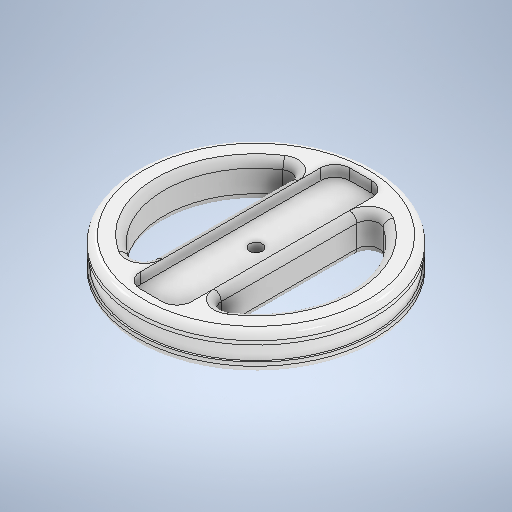
# Autodesk Inventor part: roue
Saved by Autodesk Inventor 2025 (Build 290162000, 162)
## iProperties
Created: 2024-09-05
Part Number: roue
Material: Générique
Document SubType Name: Modeling
Designer: chass
Density: 1 g/cm^3
Appearance: Par défaut
Author: chass
## iProperties of the stored document roue_Impression 3D.ipt
Created: 2024-09-05
Part Number: roue_Impression 3D
Material: Générique
Document SubType Name: Modeling
Designer: chass
Density: 1 g/cm^3
Appearance: Par défaut
Author: chass
Autodesk Inventor part; units mm, degrees
ref_plane "YZ Plane" through (0, 0, 0) normal (1, 0, 0) x (0, 1, 0)
ref_plane "XZ Plane" through (0, 0, 0) normal (0, 1, 0) x (-1, 0, 0)
ref_plane "XY Plane" through (0, 0, 0) normal (0, 0, 1) x (1, 0, 0)
sketch "Esquisse2" plane through (0, 0, 0) normal (0, 0, 1) x (1, 0, 0)
  line L0 (0, 0) -> (32.5, 0)
  line L1 (32.5, 0) -> (32.5, -10)
  line L2 (32.5, -10) -> (0, -10)
  line L3 (0, -10) -> (0, 0)
  line L4 (32.5, -3) -> (32, -3)
  line L5 (32, -3) -> (32, -7)
  line L6 (32, -7) -> (32.5, -7)
  line L7 (32.5, -7) -> (32.5, -3)
  dimension "d1" = 32.5
  dimension "d2" = 10
  dimension "d6" = 3
  dimension "d7" = 0.5
  dimension "d13" = 3
  constraints: 16 end point, 4 parallel, 2 horizontal, 2 perpendicular, 1 coincident, 1 point on line
  measures "d1" distance of L1.end L2.end
  measures "d2" distance of L2.end L0.start
  measures "d6" distance between parallel lines of L2 L6
  measures "d7" distance of L4.start L4.end
  measures "d13" distance between parallel lines of L0 L4
revolve "Révolution1" add sketch "Esquisse2" angle 360 about axis through (0, -10, 0) along (0, 1, 0) contours L0 L1 L4 L5 L6 L2 L3
sketch "Esquisse3" plane through (0, 0, 0) normal (0, 1, 0) x (1, 0, 0)
  line L0 (-7, -28.5) -> (7, -28.5)
  line L1 (7, -28.5) -> (7, 28.5)
  line L2 (7, 28.5) -> (-7, 28.5)
  line L3 (-7, 28.5) -> (-7, -28.5)
  line L4 (-7, -28.5) -> (7, 28.5)
  line L5 (7, -28.5) -> (-7, 28.5)
  point P0 (0, 0)
  point P1 (0, 0)
  point P2 (0, 0)
  dimension "d9" = 14
  dimension "d10" = 57
  constraints: 12 end point, 2 midpoint, 2 parallel, 1 coincident, 1 horizontal, 1 perpendicular
  measures "d9" distance of L2.end L1.end
  measures "d10" distance of L1.end L0.end
extrude "Extrusion1" cut sketch "Esquisse3" against normal blind 3
fillet "Congé1" radius 4 4 edges at (-7, -1.5, -28.5) (7, -1.5, -28.5) (-7, -1.5, 28.5) (7, -1.5, 28.5)
sketch "Esquisse4" plane through (0, -3, 0) normal (0, 1, 0) x (1, 0, 0)
  circle A0 centre (0, 0) radius 1.75
  point P0 (0, 0)
  dimension "d15" = 3.5
  constraints: 1 centre point, 1 coincident
  measures "d15" diameter of A0
extrude "Extrusion2" cut sketch "Esquisse4" against normal blind 10
fillet "Congé2" radius 2 2 edges at (-32.5, 0, 0) (-32.5, -10, 0)
sketch "Esquisse5" plane through (0, 0, 0) normal (0, 1, 0) x (1, 0, 0)
  circle A0 centre (0, 0) radius 25
  line L0 (-9, 23.3238) -> (9, 23.3238)
  line L1 (9, 23.3238) -> (9, -23.3238)
  line L2 (9, -23.3238) -> (-9, -23.3238)
  line L3 (-9, -23.3238) -> (-9, 23.3238)
  dimension "d19" = 50
  dimension "d20" = 18
  constraints: 8 end point, 3 point on circle, 2 parallel, 1 centre point, 1 coincident, 1 horizontal, 1 perpendicular
  measures "d19" diameter of A0
  measures "d20" distance of L0.start L0.end
extrude "Extrusion3" cut sketch "Esquisse5" against normal blind 38.5 contours A0 L1 | L3 A0
fillet "Congé3" radius 3 4 edges at (9, -5, 23.3238) (9, -5, -23.3238) (-9, -5, -23.3238) (-9, -5, 23.3238)
fillet "Congé4" radius 2 16 edges at (-10.5698, 0, -21.0762) (-9, 0, 0) (-10.5698, 0, 21.0762) (-25, 0, 0) (-10.5698, -10, 21.0762) (-9, -10, 0) (-10.5698, -10, -21.0762) (-25, -10, 0) (10.5698, 0, 21.0762) (9, 0, 0) (10.5698, 0, -21.0762) (25, 0, 0) (10.5698, -10, -21.0762) (9, -10, 0) (10.5698, -10, 21.0762) (25, -10, 0)
